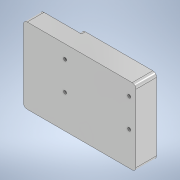
# Autodesk Inventor part: ThermalConductivityBlock
Saved by Autodesk Inventor 2021 (Build 250183000, 183)
## iProperties
Created: 2020-06-14
Part Number: ThermalConductivityBlock
Material: Generic
Document SubType Name: Modeling
Designer: Viktor Lindström
Density: 1 g/cm^3
Appearance: Default
Author: Viktor Lindström
Autodesk Inventor part; units mm, degrees
ref_plane "YZ Plane" through (0, 0, 0) normal (1, 0, 0) x (0, 1, 0)
ref_plane "XZ Plane" through (0, 0, 0) normal (0, 1, 0) x (-1, 0, 0)
ref_plane "XY Plane" through (0, 0, 0) normal (0, 0, 1) x (1, 0, 0)
sketch "Sketch1" plane through (0, 0, 0) normal (0, 0, 1) x (1, 0, 0)
  line L0 (-29.35, -19.7) -> (29.35, -19.7)
  line L1 (29.35, -19.7) -> (29.35, 19.7)
  line L2 (29.35, 19.7) -> (-29.35, 19.7)
  line L3 (-29.35, 19.7) -> (-29.35, -19.7)
  line L4 (-29.35, -19.7) -> (29.35, 19.7) construction
  line L5 (29.35, -19.7) -> (-29.35, 19.7) construction
  point P0 (0, 0)
  dimension "d0" = 39.4
  dimension "d1" = 58.7
  constraints: 12 end point, 2 midpoint, 2 parallel, 1 horizontal, 1 perpendicular
  measures "d0" distance between parallel lines of L0 L2
  measures "d1" distance between parallel lines of L1 L3
extrude "Extrusion1" add sketch "Sketch1" along normal blind 10.75
sketch "Sketch2" plane through (0, 0, 0) normal (0, 0, -1) x (-1, 0, 0)
  circle A0 centre (7.6129, -2.1018) radius 1.5 construction
  circle A1 centre (-25.8129, -2.1018) radius 1.5 construction
  circle A2 centre (-25.8129, 12.8018) radius 1.5 construction
  circle A3 centre (7.6129, 12.8018) radius 1.5 construction
  circle A4 centre (7.6129, -2.1018) radius 0.8
  circle A5 centre (-25.8129, -2.1018) radius 0.8
  circle A6 centre (-25.8129, 12.8018) radius 0.8
  circle A7 centre (7.6129, 12.8018) radius 0.8
  point P0 (0, 0)
  dimension "d4" = 1.6
  dimension "d5" = 1.6
  dimension "d6" = 1.6
  dimension "d7" = 1.6
  constraints: 4 centre point, 4 coincident
  measures "d4" diameter of A4
  measures "d5" diameter of A5
  measures "d6" diameter of A7
  measures "d7" diameter of A6
extrude "Extrusion2" cut sketch "Sketch2" against normal through all
sketch "Sketch5" plane through (0, 0, 0) normal (0, 0, -1) x (-1, 0, 0)
  line L0 (-29.35, 19.7) -> (29.35, 19.7) projected
  line L1 (29.35, -19.7) -> (9.8, -19.7)
  line L2 (9.8, -19.7) -> (9.8, 19.7)
  line L3 (9.8, 19.7) -> (29.35, 19.7)
  line L4 (29.35, 19.7) -> (29.35, -19.7)
  point P0 (0, 0)
  dimension "d10" = 19.55
  constraints: 8 end point, 2 parallel, 1 horizontal, 1 perpendicular, 1 point on line, 1 other
  measures "d10" distance between parallel lines of L4 L2
extrude "Extrusion3" cut sketch "Sketch5" against normal blind 2
fillet "Fillet1" radius 2 4 edges at (-29.35, -19.7, 6.375) (-29.35, 19.7, 6.375) (29.35, 19.7, 5.375) (29.35, -19.7, 5.375)
fillet "Fillet2" radius 2 2 edges at (-9.8, 19.7, 1) (-9.8, -19.7, 1)
equation "\"d5\" = d4"
equation "\"d6\" = d4"
equation "\"d7\" = d4"
body "Solid1"
